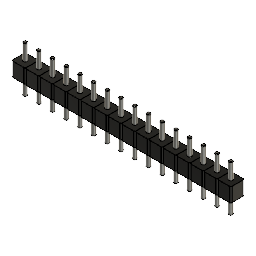
LCD+1602+I2C+v7 (Autodesk Fusion 360 archive; units mm, degrees)
design "Hřebínek"
Autodesk Fusion 360 part; units mm, degrees
sketch "Sketch1" plane through (0, 0, 0) normal (0, 0, 1) x (1, 0, 0)
  line L0 (-1, 1.25) -> (1, 1.25)
  line L1 (1.25, 1) -> (1.25, -1)
  line L2 (1, -1.25) -> (-1, -1.25)
  line L3 (-1.25, -1) -> (-1.25, 1)
  arc A0 (-1, 1.25) -> (-1.25, 1) centre (-1, 1) ccw
  arc A1 (1.25, 1) -> (1, 1.25) centre (1, 1) ccw
  arc A2 (1, -1.25) -> (1.25, -1) centre (1, -1) ccw
  arc A3 (-1.25, -1) -> (-1, -1.25) centre (-1, -1) ccw
  circle A4 centre (0, 0) radius 0.35
  dimension "d6" = 1.25
  dimension "d8" = 1.25
  dimension "d10" = 0.5
  dimension "d11" = 0.25
  dimension "d12" = 0.25
  dimension "d13" = 0.25
  dimension "d14" = 0.25
  dimension "d15" = 0.25
  dimension "d16" = 0.25
  dimension "d17" = 0.5
  dimension "d18" = 0.5
  dimension "d19" = 0.5
  dimension "d20" = 0.25
  dimension "d21" = 0.25
  dimension "d22" = 2.5
  dimension "d23" = 2.5
  dimension "d24" = 0.7
  constraint horizontal L0
  constraint vertical L1
  constraint horizontal L2
  constraint vertical L3
  constraint coincident A4.centre origin
  measures "d6" distance of A4.centre L0
  measures "d8" distance of A4.centre L3
  measures "d10" diameter of A1
  measures "d11" distance of L1 A1.centre
  measures "d12" distance of L0 A1.centre
  measures "d13" distance of L1 A2.centre
  measures "d14" distance of L2 A2.centre
  measures "d15" distance of L2 A3.centre
  measures "d16" distance of L3 A3.centre
  measures "d17" diameter of A3
  measures "d18" diameter of A2
  measures "d19" diameter of A0
  measures "d20" distance of L0 A0.centre
  measures "d21" distance of L3 A0.centre
  measures "d22" distance of L1 L3
  measures "d23" distance of L0 L2
  measures "d24" diameter of A4
extrude "Extrude1" add sketch "Sketch1" along normal blind 2.6 makes body 1
pattern_linear "R-Pattern1" count 16 spacing 2.5 along (1, 0, 0) of "Extrude1" makes body 2 at (2.4913, -0.9497, 0) makes body 3 at (5.0087, -0.9497, 0) makes body 4 at (7.5087, -0.9497, 0) makes body 5 at (10.0087, -0.9497, 0) makes body 6 at (12.5087, -0.9497, 0) makes body 7 at (15.0087, -0.9497, 0) makes body 8 at (17.4913, -0.9497, 0) makes body 9 at (19.9913, -0.9497, 0) makes body 10 at (22.4913, -0.9497, 0) makes body 11 at (24.9913, -0.9497, 0) makes body 12 at (27.4913, -0.9497, 0) makes body 13 at (29.9913, -0.9497, 0) makes body 14 at (32.4913, -0.9497, 0) makes body 15 at (34.9913, -0.9497, 0) makes body 16 at (37.4913, -0.9497, 0)
ref_plane "WorkPlane1" through (0, 0, 1.3) normal (0, 0, 1) x (1, 0, 0)
sketch "Sketch2" plane through (0, 0, 1.3) normal (0, 0, 1) x (1, 0, 0)
  circle A0 centre (0, 0) radius 0.35
  constraint coincident A0.centre origin
extrude "Extrude2" add sketch "Sketch2" along normal mid plane 8.5 separate body makes body 17
chamfer "Chamfer1" distance 0.1 angle 45 2 edges at (-0.3263, -0.1266, 5.55) (-0.3263, 0.1266, -2.95) on bodies 17
pattern_linear "R-Pattern2" count 16 spacing 2.5 along (1, 0, 0) of bodies 17 makes body 18 at (2.8483, -0.0348, 4.0667) makes body 19 at (5.3483, -0.0348, 4.0667) makes body 20 at (7.8483, -0.0348, 4.0667) makes body 21 at (9.9913, 0.3499, 4.0667) makes body 22 at (12.4913, 0.3499, 4.0667) makes body 23 at (14.9913, 0.3499, 4.0667) makes body 24 at (17.644, 0.319, 4.0667) makes body 25 at (20.144, 0.319, 4.0667) makes body 26 at (22.644, 0.319, 4.0667) makes body 27 at (25.144, 0.319, 4.0667) makes body 28 at (27.644, 0.319, 4.0667) makes body 29 at (30.144, 0.319, 4.0667) makes body 30 at (32.7043, 0.2842, 4.0667) makes body 31 at (35.2043, 0.2842, 4.0667) makes body 32 at (37.7043, 0.2842, 4.0667)
equation "POCET = 16"
equation "DISTANCE_V = 2.6 mm"
equation "DELKA_KOLIKU = 8.5 mm"
equation "PRUMER_PINU = 0.7 mm"
equation "ROZTEC_PINU = 2.5 mm"
equation "d6 = ROZTEC_PINU / 2"
equation "d8 = ROZTEC_PINU / 2"
equation "d22 = ROZTEC_PINU"
equation "d23 = ROZTEC_PINU"
equation "d24 = PRUMER_PINU"
equation "d25 = DISTANCE_V"
equation "d27 = POCET"
equation "d29 = ROZTEC_PINU"
equation "d31 = DISTANCE_V / 2"
equation "d32 = DELKA_KOLIKU / 2"
equation "d35 = POCET"
equation "d37 = ROZTEC_PINU"
